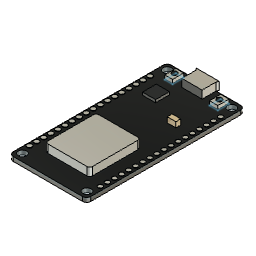
visualisation without paraglider (Autodesk Fusion 360 archive; units mm, degrees)
design "ESP32 Board - community model"
Autodesk Fusion 360 part; units mm, degrees
sketch "Sketch1" plane through (0, 0, 0) normal (0, 0, 1) x (1, 0, 0)
  line L0 (-27.7679, 28.1041) -> (-2.7247, 28.1041)
  line L1 (-1.2247, 26.6041) -> (-1.2247, -27.5391)
  line L2 (-2.7247, -29.0391) -> (-27.7679, -29.0391)
  line L3 (-29.2679, -27.5391) -> (-29.2679, 26.6041)
  arc A0 (-1.2247, 26.6041) -> (-2.7247, 28.1041) centre (-2.7247, 26.6041) ccw
  arc A1 (-27.7679, 28.1041) -> (-29.2679, 26.6041) centre (-27.7679, 26.6041) ccw
  arc A2 (-29.2679, -27.5391) -> (-27.7679, -29.0391) centre (-27.7679, -27.5391) ccw
  arc A3 (-2.7247, -29.0391) -> (-1.2247, -27.5391) centre (-2.7247, -27.5391) ccw
  dimension "d1" = 1.5
  constraint horizontal L0
  constraint vertical L1
  constraint horizontal L2
  constraint vertical L3
  constraint tangent L0 A0
  constraint tangent L1 A0
  constraint tangent L0 A1
  constraint tangent L3 A1
  constraint equal A0 A1
  constraint tangent L2 A2
  constraint tangent L3 A2
  constraint equal A0 A2
  constraint tangent L1 A3
  constraint tangent L2 A3
  constraint equal A0 A3
  measures "d1" radius of A0
extrude "Extrude1" add sketch "Sketch1" along normal blind 1.12 makes body 1
sketch "Sketch2" plane through (0, 0, 1.12) normal (0, 0, 1) x (-1, 0, 0)
  arc A0 (29.2679, 27.5391) -> (27.7679, 29.0391) centre (27.7679, 27.5391) ccw
  line L0 (27.7679, 29.0391) -> (2.7247, 29.0391)
  arc A1 (2.7247, 29.0391) -> (1.2247, 27.5391) centre (2.7247, 27.5391) ccw
  line L1 (1.2247, 27.5391) -> (1.2247, -26.6041)
  arc A2 (1.2247, -26.6041) -> (2.7247, -28.1041) centre (2.7247, -26.6041) ccw
  line L2 (2.7247, -28.1041) -> (27.7679, -28.1041)
  arc A3 (27.7679, -28.1041) -> (29.2679, -26.6041) centre (27.7679, -26.6041) ccw
  line L3 (29.2679, -26.6041) -> (29.2679, 27.5391)
  circle A4 centre (27.0863, 26.3996) radius 1.5
  circle A5 centre (3.5893, 26.5536) radius 1.5
  circle A6 centre (26.963, -25.854) radius 1.5
  circle A7 centre (3.5217, -25.7161) radius 1.5
  dimension "d4" = 3
  dimension "d5" = 3
  dimension "d6" = 3
  dimension "d7" = 3
  measures "d4" diameter of A4
  measures "d5" diameter of A5
  measures "d6" diameter of A6
  measures "d7" diameter of A7
extrude "Extrude2" cut sketch "Sketch2" against normal blind 3 contours A4 | A5 | A6 | A7 bodies 1
sketch "Sketch3" plane through (0, 0, 1.12) normal (0, 0, 1) x (-1, 0, 0)
  circle A0 centre (3.5893, 26.5536) radius 1.5
  circle A1 centre (27.0863, 26.3996) radius 1.5
  circle A2 centre (3.5217, -25.7161) radius 1.5
  circle A3 centre (26.963, -25.854) radius 1.5
  arc A4 (29.2679, 27.5391) -> (27.7679, 29.0391) centre (27.7679, 27.5391) ccw
  line L0 (27.7679, 29.0391) -> (2.7247, 29.0391)
  arc A5 (2.7247, 29.0391) -> (1.2247, 27.5391) centre (2.7247, 27.5391) ccw
  line L1 (1.2247, 27.5391) -> (1.2247, -26.6041)
  arc A6 (1.2247, -26.6041) -> (2.7247, -28.1041) centre (2.7247, -26.6041) ccw
  line L2 (2.7247, -28.1041) -> (27.7679, -28.1041)
  arc A7 (27.7679, -28.1041) -> (29.2679, -26.6041) centre (27.7679, -26.6041) ccw
  line L3 (29.2679, -26.6041) -> (29.2679, 27.5391)
  line L4 (22.4198, 3.4035) -> (8.3915, 3.4035)
  line L5 (7.3915, 4.4035) -> (7.3915, 20.7761)
  line L6 (8.3915, 21.7761) -> (22.4198, 21.7761)
  line L7 (23.4198, 20.7761) -> (23.4198, 4.4035)
  arc A8 (22.4198, 3.4035) -> (23.4198, 4.4035) centre (22.4198, 4.4035) ccw
  arc A9 (7.3915, 4.4035) -> (8.3915, 3.4035) centre (8.3915, 4.4035) ccw
  arc A10 (8.3915, 21.7761) -> (7.3915, 20.7761) centre (8.3915, 20.7761) ccw
  arc A11 (23.4198, 20.7761) -> (22.4198, 21.7761) centre (22.4198, 20.7761) ccw
  dimension "d10" = 1
  dimension "d11" = 1
  dimension "d12" = 1
  constraint horizontal L4
  constraint vertical L5
  constraint horizontal L6
  constraint vertical L7
  constraint tangent L4 A8
  constraint tangent L7 A8
  constraint tangent L4 A9
  constraint tangent L5 A9
  constraint tangent L5 A10
  constraint tangent L6 A10
  constraint tangent L6 A11
  constraint tangent L7 A11
  constraint equal A10 A11
  measures "d10" radius of A8
  measures "d11" radius of A9
  measures "d12" radius of A10
extrude "Extrude3" add sketch "Sketch3" along normal blind 3.35 contours L4 L5 L6 L7 A8 A9 A10 A11 bodies 1
sketch "Sketch4" plane through (0, 0, 1.12) normal (0, 0, 1) x (-1, 0, 0)
  line L0 (22.4198, 3.4035) -> (8.3915, 3.4035)
  arc A0 (7.3915, 4.4035) -> (8.3915, 3.4035) centre (8.3915, 4.4035) ccw
  line L1 (7.3915, 4.4035) -> (7.3915, 20.7761)
  arc A1 (8.3915, 21.7761) -> (7.3915, 20.7761) centre (8.3915, 20.7761) ccw
  line L2 (8.3915, 21.7761) -> (22.4198, 21.7761)
  arc A2 (23.4198, 20.7761) -> (22.4198, 21.7761) centre (22.4198, 20.7761) ccw
  line L3 (23.4198, 20.7761) -> (23.4198, 4.4035)
  arc A3 (22.4198, 3.4035) -> (23.4198, 4.4035) centre (22.4198, 4.4035) ccw
  circle A4 centre (3.5893, 26.5536) radius 1.5
  circle A5 centre (27.0863, 26.3996) radius 1.5
  circle A6 centre (3.5217, -25.7161) radius 1.5
  circle A7 centre (26.963, -25.854) radius 1.5
  arc A8 (29.2679, 27.5391) -> (27.7679, 29.0391) centre (27.7679, 27.5391) ccw
  line L4 (27.7679, 29.0391) -> (2.7247, 29.0391)
  arc A9 (2.7247, 29.0391) -> (1.2247, 27.5391) centre (2.7247, 27.5391) ccw
  line L5 (1.2247, 27.5391) -> (1.2247, -26.6041)
  arc A10 (1.2247, -26.6041) -> (2.7247, -28.1041) centre (2.7247, -26.6041) ccw
  line L6 (2.7247, -28.1041) -> (27.7679, -28.1041)
  arc A11 (27.7679, -28.1041) -> (29.2679, -26.6041) centre (27.7679, -26.6041) ccw
  line L7 (29.2679, -26.6041) -> (29.2679, 27.5391)
  line L8 (24.8453, -26.822) -> (22.0077, -26.822)
  line L9 (22.0077, -26.822) -> (22.0077, -22.7873)
  line L10 (22.0077, -22.7873) -> (24.8453, -22.7873)
  line L11 (24.8453, -22.7873) -> (24.8453, -26.822)
  line L12 (8.6622, -26.822) -> (5.6473, -26.822)
  line L13 (5.6473, -26.822) -> (5.6473, -22.7873)
  line L14 (5.6473, -22.7873) -> (8.6622, -22.7873)
  line L15 (8.6622, -22.7873) -> (8.6622, -26.822)
  constraint horizontal L8
  constraint vertical L9
  constraint horizontal L10
  constraint vertical L11
  constraint horizontal L12
  constraint vertical L13
  constraint horizontal L14
  constraint vertical L15
extrude "Extrude4" add sketch "Sketch4" 1 faces at (-12.9587, 15.2737, 1.12) along normal blind 0.4 contours L8 L9 L10 L11 | L12 L13 L14 L15 on bodies 1 bodies 1
extrude "Extrude5" add sketch "Sketch4" along normal blind 1.5 separate body contours L8 L9 L10 L11 | L12 L13 L14 L15 makes body 2 at (-23.8994, 25.4771, 1.12) makes body 3 at (-7.6573, 25.4771, 1.12)
sketch "Sketch5" plane through (0, 0, 2.62) normal (0, 0, 1) x (-1, 0, 0)
  line L0 (24.8453, -22.7873) -> (22.0077, -22.7873)
  line L1 (22.0077, -22.7873) -> (22.0077, -26.822)
  line L2 (22.0077, -26.822) -> (24.8453, -26.822)
  line L3 (24.8453, -26.822) -> (24.8453, -22.7873)
  circle A0 centre (23.4803, -24.9857) radius 0.9069
extrude "Extrude6" add sketch "Sketch5" along normal blind 0.2 contours A0 bodies 2
sketch "Sketch6" plane through (0, 0, 2.62) normal (0, 0, 1) x (-1, 0, 0)
  line L0 (8.6622, -22.7873) -> (5.6473, -22.7873)
  line L1 (5.6473, -22.7873) -> (5.6473, -26.822)
  line L2 (5.6473, -26.822) -> (8.6622, -26.822)
  line L3 (8.6622, -26.822) -> (8.6622, -22.7873)
  circle A0 centre (7.1404, -24.8458) radius 0.9007
extrude "Extrude7" add sketch "Sketch6" along normal blind 0.2 contours A0 bodies 3
sketch "Sketch7" plane through (0, 0, 1.52) normal (0, 0, 1) x (-1, 0, 0)
  line L0 (22.4198, 3.4035) -> (8.3915, 3.4035)
  arc A0 (7.3915, 4.4035) -> (8.3915, 3.4035) centre (8.3915, 4.4035) ccw
  line L1 (7.3915, 4.4035) -> (7.3915, 20.7761)
  arc A1 (8.3915, 21.7761) -> (7.3915, 20.7761) centre (8.3915, 20.7761) ccw
  line L2 (8.3915, 21.7761) -> (22.4198, 21.7761)
  arc A2 (23.4198, 20.7761) -> (22.4198, 21.7761) centre (22.4198, 20.7761) ccw
  line L3 (23.4198, 20.7761) -> (23.4198, 4.4035)
  arc A3 (22.4198, 3.4035) -> (23.4198, 4.4035) centre (22.4198, 4.4035) ccw
  circle A4 centre (3.5893, 26.5536) radius 1.5
  circle A5 centre (27.0863, 26.3996) radius 1.5
  circle A6 centre (3.5217, -25.7161) radius 1.5
  circle A7 centre (26.963, -25.854) radius 1.5
  arc A8 (29.2679, 27.5391) -> (27.7679, 29.0391) centre (27.7679, 27.5391) ccw
  line L4 (27.7679, 29.0391) -> (2.7247, 29.0391)
  arc A9 (2.7247, 29.0391) -> (1.2247, 27.5391) centre (2.7247, 27.5391) ccw
  line L5 (1.2247, 27.5391) -> (1.2247, -26.6041)
  arc A10 (1.2247, -26.6041) -> (2.7247, -28.1041) centre (2.7247, -26.6041) ccw
  line L6 (2.7247, -28.1041) -> (27.7679, -28.1041)
  arc A11 (27.7679, -28.1041) -> (29.2679, -26.6041) centre (27.7679, -26.6041) ccw
  line L7 (29.2679, -26.6041) -> (29.2679, 27.5391)
  line L8 (10.4946, -11.1236) -> (7.369, -11.1236)
  line L9 (7.369, -11.1236) -> (7.369, -9.3347)
  line L10 (7.369, -9.3347) -> (10.4946, -9.3347)
  line L11 (10.4946, -9.3347) -> (10.4946, -11.1236)
  dimension "d23" = 3.1255
  constraint horizontal L8
  constraint vertical L9
  constraint horizontal L10
  constraint vertical L11
  measures "d23" distance of L8.start L8.end
extrude "Extrude8" add sketch "Sketch7" along normal blind 1.9 contours L8 L9 L10 L11 bodies 1
sketch "Sketch8" plane through (0, 0, 1.52) normal (0, 0, 1) x (-1, 0, 0)
  line L0 (10.4946, -9.3347) -> (10.4946, -11.1236)
  line L1 (10.4946, -11.1236) -> (7.369, -11.1236)
  line L2 (7.369, -11.1236) -> (7.369, -9.3347)
  line L3 (7.369, -9.3347) -> (10.4946, -9.3347)
  line L4 (22.4198, 3.4035) -> (8.3915, 3.4035)
  arc A0 (7.3915, 4.4035) -> (8.3915, 3.4035) centre (8.3915, 4.4035) ccw
  line L5 (7.3915, 4.4035) -> (7.3915, 20.7761)
  arc A1 (8.3915, 21.7761) -> (7.3915, 20.7761) centre (8.3915, 20.7761) ccw
  line L6 (8.3915, 21.7761) -> (22.4198, 21.7761)
  arc A2 (23.4198, 20.7761) -> (22.4198, 21.7761) centre (22.4198, 20.7761) ccw
  line L7 (23.4198, 20.7761) -> (23.4198, 4.4035)
  arc A3 (22.4198, 3.4035) -> (23.4198, 4.4035) centre (22.4198, 4.4035) ccw
  circle A4 centre (3.5893, 26.5536) radius 1.5
  circle A5 centre (27.0863, 26.3996) radius 1.5
  circle A6 centre (3.5217, -25.7161) radius 1.5
  circle A7 centre (26.963, -25.854) radius 1.5
  arc A8 (29.2679, 27.5391) -> (27.7679, 29.0391) centre (27.7679, 27.5391) ccw
  line L8 (27.7679, 29.0391) -> (2.7247, 29.0391)
  arc A9 (2.7247, 29.0391) -> (1.2247, 27.5391) centre (2.7247, 27.5391) ccw
  line L9 (1.2247, 27.5391) -> (1.2247, -26.6041)
  arc A10 (1.2247, -26.6041) -> (2.7247, -28.1041) centre (2.7247, -26.6041) ccw
  line L10 (2.7247, -28.1041) -> (27.7679, -28.1041)
  arc A11 (27.7679, -28.1041) -> (29.2679, -26.6041) centre (27.7679, -26.6041) ccw
  line L11 (29.2679, -26.6041) -> (29.2679, 27.5391)
  line L12 (18.9374, -28.1041) -> (11.6088, -28.1041)
  line L13 (11.6088, -28.1041) -> (11.6088, -23.0647)
  line L14 (11.6088, -23.0647) -> (18.9374, -23.0647)
  line L15 (18.9374, -23.0647) -> (18.9374, -28.1041)
  line L16 (11.6088, -28.1041) -> (11.2566, -28.89)
  line L17 (11.2566, -28.89) -> (19.5385, -28.89)
  line L18 (19.5385, -28.89) -> (18.9374, -28.1041)
  constraint horizontal L12
  constraint vertical L13
  constraint horizontal L14
  constraint vertical L15
  constraint coincident L10 L12.start
  constraint perpendicular L13 L17
extrude "Extrude9" add sketch "Sketch8" along normal blind 2.83 contours L10 L12 L16 L17 L18 | L10 L12 L13 L14 L15 bodies 1
sketch "Sketch9" plane through (0, 0, 1.52) normal (0, 0, 1) x (-1, 0, 0)
  line L0 (18.9374, -23.0647) -> (18.9374, -28.1041)
  line L1 (18.9374, -28.1041) -> (27.7679, -28.1041)
  arc A0 (27.7679, -28.1041) -> (29.2679, -26.6041) centre (27.7679, -26.6041) ccw
  line L2 (29.2679, -26.6041) -> (29.2679, 27.5391)
  arc A1 (29.2679, 27.5391) -> (27.7679, 29.0391) centre (27.7679, 27.5391) ccw
  line L3 (27.7679, 29.0391) -> (2.7247, 29.0391)
  arc A2 (2.7247, 29.0391) -> (1.2247, 27.5391) centre (2.7247, 27.5391) ccw
  line L4 (1.2247, 27.5391) -> (1.2247, -26.6041)
  arc A3 (1.2247, -26.6041) -> (2.7247, -28.1041) centre (2.7247, -26.6041) ccw
  line L5 (2.7247, -28.1041) -> (11.6088, -28.1041)
  line L6 (11.6088, -28.1041) -> (11.6088, -23.0647)
  line L7 (11.6088, -23.0647) -> (18.9374, -23.0647)
  line L8 (10.4946, -9.3347) -> (10.4946, -11.1236)
  line L9 (10.4946, -11.1236) -> (7.369, -11.1236)
  line L10 (7.369, -11.1236) -> (7.369, -9.3347)
  line L11 (7.369, -9.3347) -> (10.4946, -9.3347)
  line L12 (22.4198, 3.4035) -> (8.3915, 3.4035)
  arc A4 (7.3915, 4.4035) -> (8.3915, 3.4035) centre (8.3915, 4.4035) ccw
  line L13 (7.3915, 4.4035) -> (7.3915, 20.7761)
  arc A5 (8.3915, 21.7761) -> (7.3915, 20.7761) centre (8.3915, 20.7761) ccw
  line L14 (8.3915, 21.7761) -> (22.4198, 21.7761)
  arc A6 (23.4198, 20.7761) -> (22.4198, 21.7761) centre (22.4198, 20.7761) ccw
  line L15 (23.4198, 20.7761) -> (23.4198, 4.4035)
  arc A7 (22.4198, 3.4035) -> (23.4198, 4.4035) centre (22.4198, 4.4035) ccw
  circle A8 centre (3.5893, 26.5536) radius 1.5
  circle A9 centre (27.0863, 26.3996) radius 1.5
  circle A10 centre (3.5217, -25.7161) radius 1.5
  circle A11 centre (26.963, -25.854) radius 1.5
  line L16 (23.5872, -18.4953) -> (18.8554, -18.4953)
  line L17 (18.8554, -18.4953) -> (18.8554, -13.4916)
  line L18 (18.8554, -13.4916) -> (23.5872, -13.4916)
  line L19 (23.5872, -13.4916) -> (23.5872, -18.4953)
  constraint horizontal L16
  constraint vertical L17
  constraint horizontal L18
  constraint vertical L19
extrude "Extrude10" add sketch "Sketch9" along normal blind 1 contours L16 L17 L18 L19 bodies 1
sketch "Sketch10" plane through (0, 0, 1.52) normal (0, 0, 1) x (-1, 0, 0)
  line L0 (23.5872, -13.4916) -> (23.5872, -18.4953)
  line L1 (23.5872, -18.4953) -> (18.8554, -18.4953)
  line L2 (18.8554, -18.4953) -> (18.8554, -13.4916)
  line L3 (18.8554, -13.4916) -> (23.5872, -13.4916)
  line L4 (18.9374, -23.0647) -> (18.9374, -28.1041)
  line L5 (18.9374, -28.1041) -> (27.7679, -28.1041)
  arc A0 (27.7679, -28.1041) -> (29.2679, -26.6041) centre (27.7679, -26.6041) ccw
  line L6 (29.2679, -26.6041) -> (29.2679, 27.5391)
  arc A1 (29.2679, 27.5391) -> (27.7679, 29.0391) centre (27.7679, 27.5391) ccw
  line L7 (27.7679, 29.0391) -> (2.7247, 29.0391)
  arc A2 (2.7247, 29.0391) -> (1.2247, 27.5391) centre (2.7247, 27.5391) ccw
  line L8 (1.2247, 27.5391) -> (1.2247, -26.6041)
  arc A3 (1.2247, -26.6041) -> (2.7247, -28.1041) centre (2.7247, -26.6041) ccw
  line L9 (2.7247, -28.1041) -> (11.6088, -28.1041)
  line L10 (11.6088, -28.1041) -> (11.6088, -23.0647)
  line L11 (11.6088, -23.0647) -> (18.9374, -23.0647)
  line L12 (10.4946, -9.3347) -> (10.4946, -11.1236)
  line L13 (10.4946, -11.1236) -> (7.369, -11.1236)
  line L14 (7.369, -11.1236) -> (7.369, -9.3347)
  line L15 (7.369, -9.3347) -> (10.4946, -9.3347)
  line L16 (22.4198, 3.4035) -> (8.3915, 3.4035)
  arc A4 (7.3915, 4.4035) -> (8.3915, 3.4035) centre (8.3915, 4.4035) ccw
  line L17 (7.3915, 4.4035) -> (7.3915, 20.7761)
  arc A5 (8.3915, 21.7761) -> (7.3915, 20.7761) centre (8.3915, 20.7761) ccw
  line L18 (8.3915, 21.7761) -> (22.4198, 21.7761)
  arc A6 (23.4198, 20.7761) -> (22.4198, 21.7761) centre (22.4198, 20.7761) ccw
  line L19 (23.4198, 20.7761) -> (23.4198, 4.4035)
  arc A7 (22.4198, 3.4035) -> (23.4198, 4.4035) centre (22.4198, 4.4035) ccw
  circle A8 centre (3.5893, 26.5536) radius 1.5
  circle A9 centre (27.0863, 26.3996) radius 1.5
  circle A10 centre (3.5217, -25.7161) radius 1.5
  circle A11 centre (26.963, -25.854) radius 1.5
  circle A12 centre (2.5537, -20.7392) radius 0.827
  dimension "d30" = 1.654
  measures "d30" diameter of A12
extrude "Extrude11" add sketch "Sketch10" along normal blind 0.2 contours A12 bodies 1
pattern_linear "R-Pattern1" count 18 spacing 2.5588 along (0, -1, 0) of 2 faces at (-2.2986, 20.4643, 1.72) (-3.3766, 20.8215, 1.5867) on bodies 1
sketch "Sketch11" plane through (0, 0, 1.52) normal (0, 0, 1) x (-1, 0, 0)
  circle A0 centre (2.5537, 22.7608) radius 0.827
  circle A1 centre (2.5537, 20.202) radius 0.827
  circle A2 centre (2.5537, 17.6432) radius 0.827
  circle A3 centre (2.5537, 15.0843) radius 0.827
  circle A4 centre (2.5537, 12.5255) radius 0.827
  circle A5 centre (2.5537, 9.9667) radius 0.827
  circle A6 centre (2.5537, 7.4079) radius 0.827
  circle A7 centre (2.5537, 4.8491) radius 0.827
  circle A8 centre (2.5537, 2.2902) radius 0.827
  circle A9 centre (2.5537, -0.2686) radius 0.827
  circle A10 centre (2.5537, -2.8274) radius 0.827
  circle A11 centre (2.5537, -5.3862) radius 0.827
  circle A12 centre (2.5537, -7.9451) radius 0.827
  circle A13 centre (2.5537, -10.5039) radius 0.827
  circle A14 centre (2.5537, -13.0627) radius 0.827
  circle A15 centre (2.5537, -15.6215) radius 0.827
  circle A16 centre (2.5537, -18.1804) radius 0.827
  circle A17 centre (2.5537, -20.7392) radius 0.827
  line L0 (23.5872, -13.4916) -> (23.5872, -18.4953)
  line L1 (23.5872, -18.4953) -> (18.8554, -18.4953)
  line L2 (18.8554, -18.4953) -> (18.8554, -13.4916)
  line L3 (18.8554, -13.4916) -> (23.5872, -13.4916)
  line L4 (18.9374, -23.0647) -> (18.9374, -28.1041)
  line L5 (18.9374, -28.1041) -> (27.7679, -28.1041)
  arc A18 (27.7679, -28.1041) -> (29.2679, -26.6041) centre (27.7679, -26.6041) ccw
  line L6 (29.2679, -26.6041) -> (29.2679, 27.5391)
  arc A19 (29.2679, 27.5391) -> (27.7679, 29.0391) centre (27.7679, 27.5391) ccw
  line L7 (27.7679, 29.0391) -> (2.7247, 29.0391)
  arc A20 (2.7247, 29.0391) -> (1.2247, 27.5391) centre (2.7247, 27.5391) ccw
  line L8 (1.2247, 27.5391) -> (1.2247, -26.6041)
  arc A21 (1.2247, -26.6041) -> (2.7247, -28.1041) centre (2.7247, -26.6041) ccw
  line L9 (2.7247, -28.1041) -> (11.6088, -28.1041)
  line L10 (11.6088, -28.1041) -> (11.6088, -23.0647)
  line L11 (11.6088, -23.0647) -> (18.9374, -23.0647)
  line L12 (10.4946, -9.3347) -> (10.4946, -11.1236)
  line L13 (10.4946, -11.1236) -> (7.369, -11.1236)
  line L14 (7.369, -11.1236) -> (7.369, -9.3347)
  line L15 (7.369, -9.3347) -> (10.4946, -9.3347)
  line L16 (22.4198, 3.4035) -> (8.3915, 3.4035)
  arc A22 (7.3915, 4.4035) -> (8.3915, 3.4035) centre (8.3915, 4.4035) ccw
  line L17 (7.3915, 4.4035) -> (7.3915, 20.7761)
  arc A23 (8.3915, 21.7761) -> (7.3915, 20.7761) centre (8.3915, 20.7761) ccw
  line L18 (8.3915, 21.7761) -> (22.4198, 21.7761)
  arc A24 (23.4198, 20.7761) -> (22.4198, 21.7761) centre (22.4198, 20.7761) ccw
  line L19 (23.4198, 20.7761) -> (23.4198, 4.4035)
  arc A25 (22.4198, 3.4035) -> (23.4198, 4.4035) centre (22.4198, 4.4035) ccw
  circle A26 centre (3.5893, 26.5536) radius 1.5
  circle A27 centre (27.0863, 26.3996) radius 1.5
  circle A28 centre (3.5217, -25.7161) radius 1.5
  circle A29 centre (26.963, -25.854) radius 1.5
  circle A30 centre (28.0891, -20.779) radius 0.9039
extrude "Extrude12" add sketch "Sketch11" along normal blind 0.2 contours A30 bodies 1
pattern_linear "R-Pattern2" count 18 spacing 2.5647 along (0, -1, 0) of 2 faces at (-28.4609, 19.9551, 1.6533) (-27.8177, 20.7322, 1.72) on bodies 1
